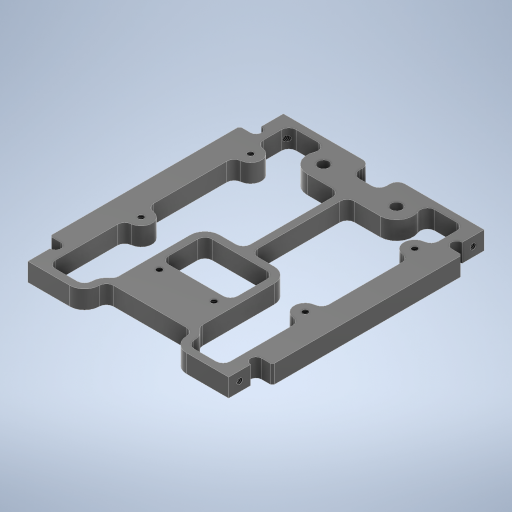
# Autodesk Inventor part: HeadCircuitMountFrame
Saved by Autodesk Inventor 2024.2 (Build 282272000, 272)
## iProperties
Created: 2024-01-19
Part Number: HeadCircuitMountFrame
Material: Acetal Resin, Black
Document SubType Name: Modeling
Designer: Masato Kubotera
Density: 1.425 g/cm^3
Appearance: Smooth - Black
Mass: 11.7532 g
Surface Area: 68.8447 cm^2
Volume: 8.24788 cm^3
Vendor: meviy
Author: Masato Kubotera
Autodesk Inventor part; units mm, degrees
ref_plane "YZ Plane" through (0, 0, 0) normal (1, 0, 0) x (0, 1, 0)
ref_plane "XZ Plane" through (0, 0, 0) normal (0, 1, 0) x (-1, 0, 0)
ref_plane "XY Plane" through (0, 0, 0) normal (0, 0, 1) x (1, 0, 0)
sketch "Sketch1" plane through (0, 0, 0) normal (0, 0, 1) x (1, 0, 0)
  line L0 (35, 27.5) -> (-35, 27.5) construction
  line L1 (-35, 27.5) -> (-35, -27.5) construction
  line L2 (-35, -27.5) -> (35, -27.5) construction
  line L3 (35, -27.5) -> (35, 27.5) construction
  line L4 (35, 27.5) -> (-35, -27.5) construction
  line L5 (-35, 27.5) -> (35, -27.5) construction
  line L6 (0, 27.5) -> (0, -27.5) construction
  line L7 (35, 0) -> (-35, 0) construction
  line L8 (26, 27.5) -> (26, 30.5)
  line L9 (26, 30.5) -> (-26, 30.5)
  line L10 (-26, 30.5) -> (-26, 27.5)
  arc A0 (-29, 27.5) -> (-26, 27.5) centre (-27.5, 27.5) ccw
  line L11 (26, -27.5) -> (26, -30.5)
  line L12 (26, -30.5) -> (-26, -30.5)
  line L13 (-26, -30.5) -> (-26, -27.5)
  arc A1 (-26, -27.5) -> (-29, -27.5) centre (-27.5, -27.5) ccw
  line L14 (-32, 27.5) -> (-32, 21.5) construction
  line L15 (0, 30.5) -> (0, 27.5) construction
  line L16 (32, 27.5) -> (32, 21.5) construction
  arc A2 (26, 27.5) -> (29, 27.5) centre (27.5, 27.5) ccw
  arc A3 (29, -27.5) -> (26, -27.5) centre (27.5, -27.5) ccw
  line L17 (26.5, -10) -> (4, -10) construction
  line L18 (4, -10) -> (4, 10) construction
  line L19 (4, 10) -> (26.5, 10) construction
  line L20 (26.5, 10) -> (26.5, -10) construction
  line L21 (26.5, -10) -> (4, 10) construction
  line L22 (4, -10) -> (26.5, 10) construction
  line L23 (19, -7.5) -> (19, 7.5) construction
  line L24 (35, -27.5) -> (35, -16)
  line L25 (29, -10) -> (29, 10)
  line L26 (35, 16) -> (35, 27.5)
  arc A4 (31, 12) -> (29, 10) centre (31, 10) ccw
  arc A5 (31, 12) -> (35, 16) centre (31, 16) ccw
  line L27 (-28.5, -10) -> (-28.5, 10) construction
  circle A6 centre (-28.5, 10) radius 2.5 construction
  line L28 (-33, 3.75) -> (-32, 3.75)
  line L29 (-30, 1.75) -> (-30, -1.75)
  line L30 (-32, -3.75) -> (-33, -3.75)
  line L31 (-35, -5.75) -> (-35, -27.5)
  line L32 (-35, 5.75) -> (-35, 27.5)
  arc A7 (-33, -3.75) -> (-35, -5.75) centre (-33, -5.75) ccw
  arc A8 (-32, -3.75) -> (-30, -1.75) centre (-32, -1.75) ccw
  arc A9 (-30, 1.75) -> (-32, 3.75) centre (-32, 1.75) ccw
  arc A10 (-35, 5.75) -> (-33, 3.75) centre (-33, 5.75) ccw
  line L33 (35, -27.5) -> (29, -27.5)
  line L34 (-29, -27.5) -> (-35, -27.5)
  line L35 (-35, 27.5) -> (-29, 27.5)
  line L36 (29, 27.5) -> (35, 27.5)
  line L37 (6.5, 9.5) -> (14.5, 9.5)
  line L38 (16.5, 7.5) -> (16.5, -7.5)
  line L39 (14.5, -9.5) -> (6.5, -9.5)
  line L40 (4.5, -7.5) -> (4.5, 7.5)
  line L41 (4.5, 9.5) -> (16.5, -9.5) construction
  line L42 (16.5, 9.5) -> (4.5, -9.5) construction
  circle A11 centre (19, 7.5) radius 2.5 construction
  line L43 (11.5, -25) -> (-23.5, -25) construction
  line L44 (-23.5, -25) -> (-23.5, 25) construction
  line L45 (-23.5, 25) -> (11.5, 25) construction
  line L46 (11.5, 25) -> (11.5, -25) construction
  line L47 (11.5, -25) -> (-23.5, 25) construction
  line L48 (-23.5, -25) -> (11.5, 25) construction
  line L49 (9, 22.5) -> (-21, 22.5) construction
  line L50 (-21, 22.5) -> (-21, -22.5) construction
  line L51 (-21, -22.5) -> (9, -22.5) construction
  line L52 (9, -22.5) -> (9, 22.5) construction
  line L53 (9, 22.5) -> (-21, -22.5) construction
  line L54 (-21, 22.5) -> (9, -22.5) construction
  circle A12 centre (-21, 22.5) radius 2.5 construction
  arc A13 (-23.985, 22.2) -> (-18.015, 22.2) centre (-21, 22.5) ccw
  line L55 (-24, 10) -> (-24, 3)
  line L56 (-16.0251, 24) -> (4.0251, 24)
  arc A14 (6.015, 22.2) -> (11.985, 22.2) centre (9, 22.5) ccw
  arc A15 (31, 14) -> (27.7511, 12.3333) centre (31, 10) ccw
  line L57 (33, 16) -> (33, 22)
  line L58 (31, 24) -> (13.9749, 24)
  arc A16 (31, 14) -> (33, 16) centre (31, 16) ccw
  line L59 (35, 16) -> (33, 16) construction
  line L60 (31, 12) -> (31, 14) construction
  line L61 (26.1266, 11.5) -> (6.5, 11.5)
  line L62 (2.5, 7.5) -> (2.5, 3)
  line L63 (0.5, 1) -> (-22, 1)
  arc A17 (26.1266, 11.5) -> (27.7511, 12.3333) centre (26.1266, 13.5) ccw
  arc A18 (33, 22) -> (31, 24) centre (31, 22) ccw
  arc A19 (13.9749, 24) -> (11.985, 22.2) centre (13.9749, 22) ccw
  arc A20 (6.015, 22.2) -> (4.0251, 24) centre (4.0251, 22) ccw
  arc A21 (-16.0251, 24) -> (-18.015, 22.2) centre (-16.0251, 22) ccw
  arc A22 (-24, 3) -> (-22, 1) centre (-22, 3) ccw
  arc A23 (0.5, 1) -> (2.5, 3) centre (0.5, 3) ccw
  arc A24 (6.5, 11.5) -> (2.5, 7.5) centre (6.5, 7.5) ccw
  arc A25 (29, -10) -> (31, -12) centre (31, -10) ccw
  arc A26 (35, -16) -> (31, -12) centre (31, -16) ccw
  arc A27 (-18.015, -22.2) -> (-23.985, -22.2) centre (-21, -22.5) ccw
  line L64 (-24, -10) -> (-24, -3)
  line L65 (-16.0251, -24) -> (4.0251, -24)
  arc A28 (11.985, -22.2) -> (6.015, -22.2) centre (9, -22.5) ccw
  arc A29 (27.7511, -12.3333) -> (31, -14) centre (31, -10) ccw
  line L66 (33, -16) -> (33, -22)
  line L67 (31, -24) -> (13.9749, -24)
  arc A30 (33, -16) -> (31, -14) centre (31, -16) ccw
  line L68 (26.1266, -11.5) -> (6.5, -11.5)
  line L69 (2.5, -7.5) -> (2.5, -3)
  line L70 (0.5, -1) -> (-22, -1)
  arc A31 (27.7511, -12.3333) -> (26.1266, -11.5) centre (26.1266, -13.5) ccw
  arc A32 (31, -24) -> (33, -22) centre (31, -22) ccw
  arc A33 (11.985, -22.2) -> (13.9749, -24) centre (13.9749, -22) ccw
  arc A34 (4.0251, -24) -> (6.015, -22.2) centre (4.0251, -22) ccw
  arc A35 (-18.015, -22.2) -> (-16.0251, -24) centre (-16.0251, -22) ccw
  arc A36 (-22, -1) -> (-24, -3) centre (-22, -3) ccw
  arc A37 (2.5, -3) -> (0.5, -1) centre (0.5, -3) ccw
  arc A38 (2.5, -7.5) -> (6.5, -11.5) centre (6.5, -7.5) ccw
  arc A39 (14.5, -9.5) -> (16.5, -7.5) centre (14.5, -7.5) ccw
  arc A40 (4.5, -7.5) -> (6.5, -9.5) centre (6.5, -7.5) ccw
  arc A41 (6.5, 9.5) -> (4.5, 7.5) centre (6.5, 7.5) ccw
  arc A42 (16.5, 7.5) -> (14.5, 9.5) centre (14.5, 7.5) ccw
  line L71 (-33, 16) -> (-33, 22)
  arc A43 (-31, 24) -> (-33, 22) centre (-31, 22) ccw
  arc A44 (-23.985, 22.2) -> (-25.9749, 24) centre (-25.9749, 22) ccw
  line L72 (-31, 24) -> (-25.9749, 24)
  arc A45 (-24, 10) -> (-30.2308, 14.1538) centre (-28.5, 10) ccw
  arc A46 (-33, 16) -> (-30.2308, 14.1538) centre (-31, 16) ccw
  line L73 (-33, -16) -> (-33, -22)
  arc A47 (-33, -22) -> (-31, -24) centre (-31, -22) ccw
  line L74 (-31, -24) -> (-25.9749, -24)
  arc A48 (-30.2308, -14.1538) -> (-24, -10) centre (-28.5, -10) ccw
  arc A49 (-30.2308, -14.1538) -> (-33, -16) centre (-31, -16) ccw
  arc A50 (-25.9749, -24) -> (-23.985, -22.2) centre (-25.9749, -22) ccw
  point P0 (0, 0)
  point P1 (0, 0)
  point P2 (0, -0.0008)
  point P3 (-29, -27.5)
  point P4 (26, -27.5)
  point P5 (-26, -27.5)
  point P6 (-26, -27.5)
  point P7 (26, -27.5)
  point P8 (15.25, 0)
  point P9 (29, -27.5)
  point P10 (10.5, 0)
  point P11 (-6, 0)
  point P12 (-35, -16.625)
  point P13 (-24, 22.5)
  point P14 (-18.4019, 24)
  point P15 (6.4019, 24)
  point P16 (11.5981, 24)
  point P17 (27.2919, 11.5)
  point P18 (30, -9.8466)
  dimension "d19" = 3
  dimension "d20" = 52
  dimension "d37" = 55
  dimension "d40" = 6
  dimension "d41" = 6
  dimension "d59" = 70
  dimension "d60" = 1.5
  dimension "d61" = 22.5
  dimension "d62" = 20
  dimension "d63" = 15
  dimension "d84" = 7.5
  dimension "d87" = 6
  dimension "d88" = 2.5
  dimension "d89" = 32.5
  dimension "d90" = 20
  dimension "d98" = 5
  dimension "d99" = 2
  dimension "d100" = 7.5
  dimension "d101" = 5
  dimension "d109" = 0.5
  dimension "d110" = 0.5
  dimension "d111" = 5
  dimension "d113" = 50
  dimension "d114" = 35
  dimension "d115" = 5
  dimension "d117" = 5
  dimension "d118" = 2
  dimension "d119" = 2
  dimension "d120" = 2
  dimension "d121" = 2
  dimension "d122" = 2
  dimension "d123" = 2
  dimension "d124" = 2
  dimension "d125" = 2
  dimension "d126" = 3
  dimension "d127" = 2
  constraints: 148 end point, 101 point on circle, 65 symmetric about line, 51 centre point, 45 tangent, 19 point on line, 17 coincident, 17 midpoint, 14 equal radius, 14 horizontal, 11 vertical, 10 parallel, 9 collinear, 5 perpendicular, 36 other
  measures "d19" distance of L8.start L8.end
  measures "d20" distance of L8.end L9.end
  measures "d37" distance of L2.end L3.end
  measures "d40" distance of L14.start L14.end
  measures "d41" distance between parallel lines of L10 L14
  measures "d59" distance of L3.end L1.start
  measures "d60" radius of A2
  measures "d61" distance of L18.end L19.end
  measures "d62" distance of L17.end L18.end
  measures "d63" distance of L23.start L23.end
  measures "d84" distance between parallel lines of L20 L23
  measures "d87" distance between parallel lines of L3 L25
  measures "d88" distance between parallel lines of L25 L20
  measures "d89" distance between parallel lines of L18 L27
  measures "d90" distance of L27.start L27.end
  measures "d98" diameter of A6
  measures "d99" radius of A7
  measures "d100" distance between parallel lines of L28 L30
  measures "d101" distance between parallel lines of L29 L1
  measures "d109" distance between parallel lines of L19 L37
  measures "d110" distance between parallel lines of L18 L40
  measures "d111" diameter of A11
  measures "d113" distance of L43.end L44.end
  measures "d114" distance of L43.start L43.end
  measures "d115" distance between parallel lines of L27 L44
  measures "d117" diameter of A12
  measures "d118" distance edge to line of A6 L55
  measures "d119" radius of A16
  measures "d120" radius of A17
  measures "d121" radius of A39
  measures "d122" distance between parallel lines of L61 L37
  measures "d123" radial gap between concentric circles of A15 A4
  measures "d124" distance edge to line of A2 L58
  measures "d125" distance between parallel lines of L63 L70
  measures "d126" radius of A14
  measures "d127" radius of A4
extrude "Extrusion1" add sketch "Sketch1" against normal blind 5
hole "M2" at (19, -7.5, 0) at (19, 7.5, 0) at (9, 22.5, 0) at (-21, 22.5, 0) at (-21, -22.5, 0) at (9, -22.5, 0) direction (0, 0, -1) diameter 1.567 end through all thread size "M2x0.4" class "6H" standard "ANSI Metric M Profile"
hole "Phi3" at (-28.5, -10, 0) at (-28.5, 10, 0) direction (0, 0, -1) diameter 3 end through all
sketch "Sketch3" plane through (29, 27.5, 0) normal (0, 1, 0) x (1, 0, 0)
  line L0 (6, 0) -> (0, 0) projected
  line L1 (3, 0) -> (3, 5)
  line L2 (-58, 0) -> (-64, 0) projected
  line L3 (-61, 0) -> (-61, 5)
  line L4 (-64, 5) -> (-58, 5) projected
  line L5 (0, 5) -> (6, 5) projected
  point P0 (-29, 0)
  point P1 (3, 0)
  point P2 (3, 2.5)
  point P3 (-61, 2.5)
  constraints: 4 end point, 4 midpoint, 2 vertical
hole "Side-M2" at (32, 27.5, -2.5) at (-32, 27.5, -2.5) direction (0, -1, 0) diameter 1.567 depth 6.3 thread size "M2x0.4" class "6H" standard "ANSI Metric M Profile"
chamfer "C0.5" distance 0.5 angle 45 4 edges at (26, -30.5, -2.5) (-26, -30.5, -2.5) (26, 30.5, -2.5) (-26, 30.5, -2.5)
mirror "Mirror1" about plane through (0, 0, 0) normal (0, 1, 0) of "Side-M2"
body "Solid1"
